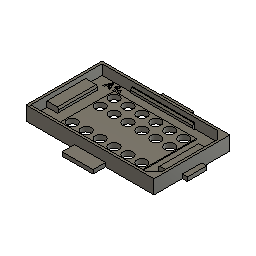
well_plate_holder (Autodesk Fusion 360 design; units mm, degrees)
Autodesk Fusion 360 part; units mm, degrees
sketch "Sketch1" plane through (0, 0, 0) normal (0, 1, 0) x (1, 0, 0)
  line L0 (79.5, 46) -> (-79.5, 46)
  line L1 (-79.5, 46) -> (-79.5, -46)
  line L2 (-79.5, -46) -> (79.5, -46)
  line L3 (79.5, -46) -> (79.5, 46)
  line L4 (79.5, 46) -> (-79.5, -46) construction
  line L5 (-79.5, 46) -> (79.5, -46) construction
  line L6 (82.5, 49) -> (-82.5, 49)
  line L7 (-82.5, 49) -> (-82.5, -49)
  line L8 (-82.5, -49) -> (82.5, -49)
  line L9 (82.5, -49) -> (82.5, 49)
  line L10 (82.5, 49) -> (-82.5, -49) construction
  line L11 (-82.5, 49) -> (82.5, -49) construction
  line L12 (-64.025, 25) -> (-64.025, -25)
  line L13 (64.025, 25) -> (64.025, -25)
  line L14 (-64.025, 0) -> (64.025, 0) construction
  line L15 (-64.025, 25) -> (-79.5, 25)
  line L16 (-64.025, -25) -> (-79.5, -25)
  line L17 (64.025, 25) -> (79.5, 25)
  line L18 (64.025, -25) -> (79.5, -25)
  line L19 (0, 43) -> (0, -43) construction
  line L20 (-40, -43) -> (40, -43)
  line L21 (-40, 43) -> (40, 43)
  line L22 (-40, 43) -> (-40, 46)
  line L23 (40, 43) -> (40, 46)
  line L24 (-40, -43) -> (-40, -46)
  line L25 (40, -43) -> (40, -46)
  line L26 (82.5, -12.5) -> (89, -12.5)
  line L27 (89, -12.5) -> (89, 12.5)
  line L28 (89, 12.5) -> (82.5, 12.5)
  line L29 (82.5, 12.5) -> (82.5, -12.5)
  line L30 (-82.5, -12.5) -> (-89, -12.5)
  line L31 (-89, -12.5) -> (-89, 12.5)
  line L32 (-89, 12.5) -> (-82.5, 12.5)
  line L33 (-82.5, 12.5) -> (-82.5, -12.5)
  line L34 (-20, 49) -> (20, 49)
  line L35 (20, 49) -> (20, 65)
  line L36 (20, 65) -> (-20, 65)
  line L37 (-20, 65) -> (-20, 49)
  line L38 (-20, -49) -> (20, -49)
  line L39 (20, -49) -> (20, -65)
  line L40 (20, -65) -> (-20, -65)
  line L41 (-20, -65) -> (-20, -49)
  circle A0 centre (-45, -27) radius 6.5
  circle A1 centre (-27, -27) radius 6.5
  circle A2 centre (-9, -27) radius 6.5
  circle A3 centre (9, -27) radius 6.5
  circle A4 centre (27, -27) radius 6.5
  circle A5 centre (45, -27) radius 6.5
  circle A6 centre (-45, -9) radius 6.5
  circle A7 centre (-27, -9) radius 6.5
  circle A8 centre (-9, -9) radius 6.5
  circle A9 centre (9, -9) radius 6.5
  circle A10 centre (27, -9) radius 6.5
  circle A11 centre (45, -9) radius 6.5
  circle A12 centre (-45, 9) radius 6.5
  circle A13 centre (-27, 9) radius 6.5
  circle A14 centre (-9, 9) radius 6.5
  circle A15 centre (9, 9) radius 6.5
  circle A16 centre (27, 9) radius 6.5
  circle A17 centre (45, 9) radius 6.5
  circle A18 centre (-45, 27) radius 6.5
  circle A19 centre (-27, 27) radius 6.5
  circle A20 centre (-9, 27) radius 6.5
  circle A21 centre (9, 27) radius 6.5
  circle A22 centre (27, 27) radius 6.5
  circle A23 centre (45, 27) radius 6.5
  line L42 (-9, 9) -> (9, -9) construction
  line L43 (-9, -9) -> (9, 9) construction
  point P0 (-64.025, 0)
  point P1 (64.025, 0)
  point P2 (0, 49)
  dimension "d3" = 3
  dimension "d4" = 3
  dimension "d11" = 128.05
  dimension "d12" = 50
  dimension "d13" = 86
  dimension "d14" = 80
  dimension "d19" = 25
  dimension "d21" = 16
  dimension "d22" = 40
  dimension "d25" = 13
  dimension "d28" = 18
  dimension "d29" = 18
  dimension "d33" = 178
  dimension "d45" = 165
  dimension "d46" = 98
  constraint horizontal L0
  constraint perpendicular L0 L1
  constraint parallel L0 L2
  constraint parallel L1 L3
  constraint coincident L4 origin
  constraint coincident L5 origin
  constraint horizontal L6
  constraint perpendicular L6 L7
  constraint parallel L6 L8
  constraint parallel L7 L9
  constraint coincident L10 origin
  constraint coincident L11 origin
  constraint parallel L1 L12
  constraint coincident L12 P0
  constraint midpoint L13 P1
  constraint midpoint L12 P0
  constraint horizontal L14
  constraint coincident origin L14
  constraint coincident P0 L14.start
  constraint coincident P1 L14.end
  constraint midpoint origin L14
  constraint equal L12 L13
  constraint coincident L1 L15.end
  constraint perpendicular L1 L15
  constraint coincident L1 L16.end
  constraint perpendicular L1 L16
  constraint coincident L3 L17.end
  constraint perpendicular L3 L17
  constraint coincident L3 L18.end
  constraint perpendicular L3 L18
  constraint vertical L19
  constraint midpoint origin L19
  constraint horizontal L20
  constraint horizontal L21
  constraint midpoint L19.start L21
  constraint midpoint L19.end L20
  constraint coincident L0 L22.end
  constraint perpendicular L0 L22
  constraint coincident L0 L23.end
  constraint perpendicular L0 L23
  constraint coincident L2 L24.end
  constraint perpendicular L2 L24
  constraint coincident L2 L25.end
  constraint perpendicular L2 L25
  constraint equal L20 L21
  constraint horizontal L26
  constraint vertical L27
  constraint horizontal L28
  constraint vertical L29
  constraint coincident L9 L26.start
  constraint symmetric L14 L26.end L27.end
  constraint horizontal L30
  constraint vertical L31
  constraint horizontal L32
  constraint vertical L33
  constraint coincident L7 L30.start
  constraint symmetric L19 L26.end L30.end
  constraint symmetric L19 L27.end L31.end
  constraint horizontal L34
  constraint vertical L35
  constraint horizontal L36
  constraint vertical L37
  constraint horizontal L38
  constraint vertical L39
  constraint horizontal L40
  constraint vertical L41
  constraint coincident L8 L38.start
  constraint midpoint L34 P2
  constraint coincident L6 P2
  constraint symmetric L14 L36.end L40.end
  constraint symmetric L14 L35.end L39.end
  constraint coincident L19 P2
  constraint coincident A14.centre L42.start
  constraint coincident A9.centre L42.end
  constraint coincident A8.centre L43.start
  constraint coincident A15.centre L43.end
  constraint coincident origin L43
  constraint coincident origin L42
  measures "d3" distance of L0 L6
  measures "d4" distance of L3 L9
  measures "d11" distance of L12 L13
  measures "d12" distance of L13.start L13.end
  measures "d13" distance of L19.start L19.end
  measures "d14" distance of L21.start L21.end
  measures "d19" distance of L26.end L27.end
  measures "d21" distance of L34.end L35.end
  measures "d22" distance of L35.end L36.end
  measures "d25" diameter of A0
  measures "d33" distance of L27 L31
  measures "d45" distance of L7 L9
  measures "d46" distance of L6 L8
extrude "Extrude1" add sketch "Sketch1" against normal blind 5 contours L0 L1 L2 L3 L12 L13 L15 L16 L17 L18 L20 L21 L22 L23 L24 L25 | L0 L21 L22 L23 | L3 L13 L17 L18 | L1 L12 L15 L16 | L2 L20 L24 L25 | L6 L7 L8 L9 L29 L33 L34 L38 | L6 L34 L35 L36 L37 | L9 L26 L27 L28 L29 | L7 L30 L31 L32 L33 | L8 L38 L39 L40 L41 | A6 | A7 | A8 | A9 | A10 | A11 makes body 1
extrude "Extrude3" add sketch "Sketch1" along normal blind 7 separate body contours L0 L21 L22 L23 | L3 L13 L17 L18 | L1 L12 L15 L16 | L2 L20 L24 L25 makes body 2 at (-13.3333, 2.3333, -43) makes body 3 at (-13.3333, 2.3333, 46) makes body 4 at (-74.3417, 0, 8.3333) makes body 5 at (69.1833, 0, -8.3333)
extrude "Extrude2" add sketch "Sketch1" along normal blind 13 contours L6 L7 L8 L9 L29 L33 L34 L38 bodies 1
chamfer "Chamfer2" distance 2 distance2 2 8 edges at (-64.025, 0, 0) (-64.025, 7, 0) (64.025, 0, 0) (64.025, 7, 0) (0, 0, 43) (0, 7, 43) (0, 0, -43) (0, 7, -43) measured on face at (-74.3417, 0, 8.3333) measured on face at (-74.3417, 7, 8.3333) measured on face at (64.025, 2.3333, -8.3333) measured on face at (69.1833, 7, -8.3333) measured on face at (13.3333, 0, 44) measured on face at (13.3333, 7, 44) measured on face at (-13.3333, 2.3333, -43) measured on face at (-13.3333, 7, -45) on bodies 2 3 4 5
combine "Combine1" operation add target body 1 tool bodies 3 2 4 5
copy_body "Body->Comp1" bodies 1 removing the originals makes body 6 in component "box bottom holder"
sketch "Sketch2" plane through (0, 0, 0) normal (0, 1, 0) x (-1, 0, 0)
  circle A0 centre (45, 27) radius 6.5
  circle A1 centre (45, -9) radius 6.5
  circle A2 centre (27, 27) radius 6.5
  circle A3 centre (27, -9) radius 6.5
  circle A4 centre (9, 27) radius 6.5
  circle A5 centre (27, -27) radius 6.5
  circle A6 centre (-27, 27) radius 6.5
  circle A7 centre (-45, -27) radius 6.5
  circle A8 centre (-9, -27) radius 6.5
  circle A9 centre (-27, -27) radius 6.5
  circle A10 centre (9, -27) radius 6.5
  circle A11 centre (-45, 27) radius 6.5
  circle A12 centre (-27, -9) radius 6.5
  circle A13 centre (-9, 27) radius 6.5
  circle A14 centre (-9, -9) radius 6.5
  circle A15 centre (9, -9) radius 6.5
  circle A16 centre (-45, -9) radius 6.5
  circle A17 centre (45, -27) radius 6.5
  line L0 (-79.5, -25) -> (-79.5, -46)
  line L1 (-79.5, -46) -> (-40, -46)
  line L2 (79.5, -46) -> (79.5, -25)
  line L3 (79.5, 46) -> (40, 46)
  line L4 (-79.5, 46) -> (-79.5, 25)
  line L5 (68.034, -38.6726) -> (56.9228, -38.6726) construction
  line L6 (56.9228, -38.6726) -> (56.9228, -44.5188) construction
  line L7 (56.9228, -44.5188) -> (68.034, -44.5188) construction
  line L8 (68.034, -44.5188) -> (68.034, -38.6726) construction
  line L9 (52.8455, -38.5007) -> (50.017, -41.3291)
  line L10 (50.017, -41.3291) -> (47.8455, -36.3291)
  line L11 (47.8455, -36.3291) -> (52.8455, -38.5007)
  line L12 (62.6062, -38.5007) -> (52.8455, -38.5007) construction
  line L13 (53, -35) -> (-53, -35)
  line L14 (-53, -35) -> (-53, 35)
  line L15 (-53, 35) -> (53, 35)
  line L16 (53, 35) -> (53, -35)
  line L17 (53, -35) -> (-53, 35) construction
  line L18 (-53, -35) -> (53, 35) construction
  line L19 (-66.025, -25) -> (-79.5, -25)
  line L20 (-40, -46) -> (-40, -45)
  line L21 (-40, -45) -> (40, -45)
  line L22 (40, -45) -> (40, -46)
  line L23 (40, -46) -> (79.5, -46)
  line L24 (79.5, -25) -> (66.025, -25)
  line L25 (66.025, -25) -> (66.025, 25)
  line L26 (66.025, 25) -> (79.5, 25)
  line L27 (79.5, 25) -> (79.5, 46)
  line L28 (40, 46) -> (40, 45)
  line L29 (40, 45) -> (-40, 45)
  line L30 (-40, 45) -> (-40, 46)
  line L31 (-40, 46) -> (-79.5, 46)
  line L32 (-79.5, 25) -> (-66.025, 25)
  line L33 (-66.025, 25) -> (-66.025, -25)
  dimension "d34" = 9
  dimension "d35" = 4
  dimension "d36" = 5
  dimension "d37" = 45
  dimension "d38" = 8
  dimension "d39" = 8
  text T0 "A1" font "Arial" height 9 bold align left top in box 11.1113 x 5.8461 at (68.034, -38.6726) x (-1, 0) y (0, -1) spacing 1 kerned
  constraint horizontal L7
  constraint equal L10 L11
  constraint horizontal L12
  constraint coincident L9.start L11.end
  constraint horizontal L13
  constraint perpendicular L13 L14
  constraint parallel L13 L15
  constraint parallel L14 L16
  constraint coincident L17 origin
  constraint coincident L18 origin
  measures "d35" distance of L9.start L9.end
  measures "d36" vertical distance of L9.end L10.end
  measures "d37" angle of L9 L12
  measures "d38" distance of A17.centre L13
  measures "d39" distance of A17.centre L16
extrude "Extrude2'" cut sketch "Sketch2" sketch "Sketch2" against normal blind 3 contours L9 L10 L11 of sketch 2 text T0 bodies 6 in component "box bottom holder"
chamfer "Chamfer1" distance 10 angle 45 2 edges at (79.5, 6.5, -46) (79.5, 6.5, 46) on bodies 6 in component "box bottom holder"
extrude "Extrude3'" add sketch "Sketch2" along normal blind 1.2 contours L13 L14 L15 L16 bodies 6 in component "box bottom holder"
component "box bottom holder" placed x (1, 0, 0) y (0, 1, 0) z (0, 0, 1) at (0, 0, 0)
equation "d11 = 127.55 mm + 0.5 mm"
equation "d13 = 85.5 mm + 0.5 mm"
